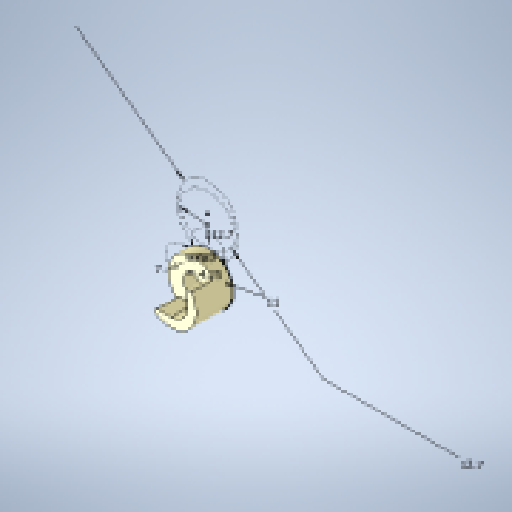
# Autodesk Inventor part: Cam - Shell
Saved by Autodesk Inventor 2023.2 (Build 272271000, 271)
## iProperties
Created: 2024-01-19
Part Number: Cam - Shell
Material: Nylon 6/6
Document SubType Name: Modeling
Designer: Nathan Cai
Density: 1.13 g/cm^3
Appearance: Nylon 6
Mass: 0.456309 g
Surface Area: 4.64642 cm^2
Volume: 0.403814 cm^3
Author: Nathan Cai
Autodesk Inventor part; units mm, degrees
ref_plane "YZ Plane" through (0, 0, 0) normal (1, 0, 0) x (0, 1, 0)
ref_plane "XZ Plane" through (0, 0, 0) normal (0, 1, 0) x (-1, 0, 0)
ref_plane "XY Plane" through (0, 0, 0) normal (0, 0, 1) x (1, 0, 0)
sketch "Sketch1" plane through (0, 0, 0) normal (0, 0, 1) x (1, 0, 0)
  circle A0 centre (0, 0) radius 2.125
  circle A1 centre (0, 0) radius 5.375
  line L0 (0, 0) -> (0, 5.375) construction
  line L1 (3.5, 0) -> (3.5, 5.375)
  line L2 (-3.5, 5.375) -> (-3.5, 0)
  arc A2 (-3.5, 0) -> (3.5, 0) centre (0, 0) ccw
  arc A3 (3.5, 5.375) -> (-3.5, 5.375) centre (0, 5.375) ccw construction
  line L3 (0, 0) -> (-5.375, 0) construction
  line L4 (0, 3.5) -> (-5.375, 3.5)
  line L5 (-5.375, -3.5) -> (0, -3.5)
  arc A4 (0, -3.5) -> (0, 3.5) centre (0, 0) ccw
  arc A5 (-5.375, 3.5) -> (-5.375, -3.5) centre (-5.375, 0) ccw construction
  circle A6 centre (0, 11.725) radius 6.35 construction
  circle A7 centre (0, 9.85) radius 6.35 construction
  arc A8 (3.5, 4.0793) -> (-4.0793, -3.5) centre (1.9038, -1.9038) ccw
  point P0 (0, 2.6875)
  point P1 (-2.6875, 0)
  point P2 (0, -3.5)
  point P3 (-4.6837, -3.75)
  point P4 (3.75, 4.6837)
  point P5 (-3.5, 4.0793)
  point P6 (-3.5, 3.5)
  point P7 (-4.0793, 3.5)
  dimension "d0" = 4.25
  dimension "d3" = 10.75
  dimension "d4" = 7
  dimension "d5" = 7
  dimension "d6" = 90
  dimension "d7" = 12.7
  dimension "d8" = 12.7
  constraints: 16 end point, 14 point on circle, 11 tangent, 9 centre point, 4 point on line, 2 coincident, 2 midpoint, 2 parallel, 1 vertical
  measures "d0" diameter of A0
  measures "d3" diameter of A1
  measures "d4" diameter of A3
  measures "d5" diameter of A5
  measures "d6" angle of L0 L3
  measures "d7" diameter of A6
  measures "d8" diameter of A7
extrude "Extrusion1" add sketch "Sketch1" along normal blind 3.175
extrude "Extrusion2" add sketch "Sketch1" along normal blind 7.9375 contours A1 L5 A2 L1
fillet "Fillet1" radius 0.5 2 edges at (3.5, 4.0793, 5.5563) (-4.0793, -3.5, 5.5563)
equation "\"d4\" = d5"
body "Solid1"
